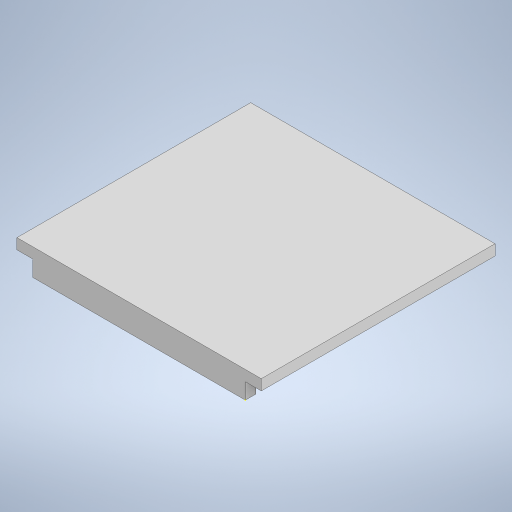
# Autodesk Inventor part: V3_O3
Saved by Autodesk Inventor 2023.1 (Build 271208000, 208)
## iProperties
Created: 2023-04-22
Part Number: V3_O3
Material: Generisch
Document SubType Name: Sheet Metal
Designer: marco
Density: 1 g/cm^3
Sheet Metal Rule: Standard_mm
Appearance: Vorgabe
Author: marco
Autodesk Inventor part; units mm, degrees
ref_plane "YZ Plane" through (0, 0, 0) normal (1, 0, 0) x (0, 1, 0)
ref_plane "XZ Plane" through (0, 0, 0) normal (0, 1, 0) x (-1, 0, 0)
ref_plane "XY Plane" through (0, 0, 0) normal (0, 0, 1) x (1, 0, 0)
sketch "Skizze1" plane through (0, 0, 0) normal (0, 1, 0) x (-1, 0, 0)
  point P0 (0, 0)
sketch "Skizze2" plane through (0, 0, 0) normal (0, 1, 0) x (-1, 0, 0)
  line L0 (0, 0) -> (20, 0)
  line L1 (20, 0) -> (20, -22)
  line L2 (20, -22) -> (0, -22)
  line L3 (0, -22) -> (0, 0)
  line L4 (0, 0) -> (20, 0)
  line L5 (20, 0) -> (20, -1)
  line L6 (20, -1) -> (0, -1)
  line L7 (0, -1) -> (0, 0)
  line L8 (0, -22) -> (20, -22)
  line L9 (20, -22) -> (20, -21)
  line L10 (20, -21) -> (0, -21)
  line L11 (0, -21) -> (0, -22)
  dimension "d0" = 20
  dimension "d1" = 22
  dimension "d2" = 20
  dimension "d3" = 1
  dimension "d4" = 20
  dimension "d5" = 1
  constraints: 24 end point, 6 parallel, 3 horizontal, 3 perpendicular
  measures "d0" distance of L1.end L2.end
  measures "d1" distance of L0.end L1.end
  measures "d2" distance of L5.end L6.end
  measures "d3" distance of L4.end L5.end
  measures "d4" distance of L10.end L9.end
  measures "d5" distance of L9.end L8.end
extrude "Extrusion1" add sketch "Skizze2" along normal blind 1.5 contours L0 L1 L6 L3 | L10 L1 L2 L3
sketch "Skizze3" plane through (0, 1.5, 0) normal (0, 1, 0) x (1, 0, 0)
  line L0 (1.5, 0) -> (-21.5, 0)
  line L1 (-21.5, 0) -> (-21.5, 22)
  line L2 (-21.5, 22) -> (1.5, 22)
  line L3 (1.5, 22) -> (1.5, 0)
  line L4 (-20, 22) -> (-20, 21) projected
  point P0 (0, 0)
  point P1 (-20, 21.5)
  dimension "d8" = 23
  dimension "d9" = 22
  dimension "d10" = 1.5
  constraints: 8 end point, 2 parallel, 1 horizontal, 1 midpoint, 1 perpendicular
  measures "d8" distance of L1.end L2.end
  measures "d9" distance of L0.end L1.end
  measures "d10" distance from line of L1 point (-20, 21.5)
extrude "Extrusion2" add sketch "Skizze3" along normal blind 1
equation "\"Biegeradius\" = Stärke"
equation "\"BreiteBiegungsfreistellung\" = Stärke"
equation "\"TiefeBiegungsfreistellung\" = 0.5 * Stärke"
equation "\"GrößeEckenfreistellung\" = 4 * Stärke"
equation "\"MinimalRest\" = 2 * Stärke"
equation "\"Übergangsradius\" = Biegeradius"
equation "\"JacobiRadiusGröße\" = Biegeradius"
equation "\"Abstandsgröße\" = Stärke"
equation "\"Stärke\" = 0.5"
